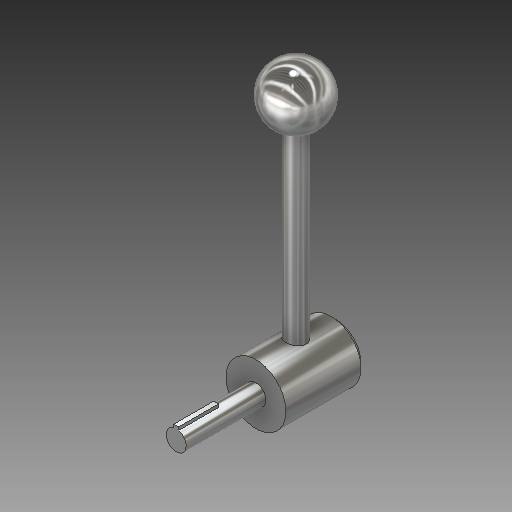
# Autodesk Inventor part: Handle
Saved by Autodesk Inventor 2018 (Build 220112000, 112)
## iProperties
Created: 2017-12-22
Part Number: Handle
Material: Stainless Steel
Document SubType Name: Modeling
Designer: 232963
Density: 8 g/cm^3
Appearance: Chrome - Polished
Author: 232963
Autodesk Inventor part; units mm, degrees
ref_plane "YZ Plane" through (0, 0, 0) normal (1, 0, 0) x (0, 1, 0)
ref_plane "XZ Plane" through (0, 0, 0) normal (0, 1, 0) x (-1, 0, 0)
ref_plane "XY Plane" through (0, 0, 0) normal (0, 0, 1) x (1, 0, 0)
sketch "Sketch1" plane through (0, 0, 0) normal (0, 0, 1) x (1, 0, 0)
  circle A0 centre (0, 0) radius 9.525
  dimension "d0" = 19.05
  constraints: 1 centre point, 1 coincident
  measures "d0" diameter of A0
extrude "Extrusion1" add sketch "Sketch1" along normal blind 25.4
sketch "Sketch2" plane through (0, 0, 25.4) normal (0, 0, 1) x (1, 0, 0)
  circle A0 centre (0, 0) radius 3.175
  dimension "d3" = 6.35
  constraints: 1 centre point, 1 coincident
  measures "d3" diameter of A0
extrude "Extrusion2" add sketch "Sketch2" along normal blind 25.4
sketch "Sketch3" plane through (0, 0, 50.8) normal (0, 0, 1) x (1, 0, 0)
  line L0 (-0.762, 4.064) -> (0.762, 4.064)
  line L1 (0.762, 4.064) -> (0.762, 2.2428)
  line L2 (0.762, 2.2428) -> (-0.762, 2.2428)
  line L3 (-0.762, 2.2428) -> (-0.762, 4.064)
  point P0 (0, 0)
  dimension "d6" = 4.064
  dimension "d7" = 0.762
  dimension "d8" = 1.524
  constraints: 8 end point, 2 parallel, 1 horizontal, 1 perpendicular
  measures "d6" distance from line of point (0, 0) L0
  measures "d7" distance from line of point (0, 0) L3
  measures "d8" distance of L0.start L0.end
extrude "Extrusion3" add sketch "Sketch3" against normal blind 12.7
sketch "Sketch4" plane through (0, 0, 0) normal (0, 1, 0) x (-1, 0, 0)
  line L0 (-9.525, 0) -> (-9.525, 25.4) projected
  line L1 (-9.525, 25.4) -> (-3.175, 25.4) projected
  line L2 (-3.175, 25.4) -> (-3.175, 50.8) projected
  line L3 (-3.175, 50.8) -> (3.175, 50.8) projected
  line L4 (3.175, 50.8) -> (3.175, 25.4) projected
  line L5 (3.175, 25.4) -> (9.525, 25.4) projected
  line L6 (9.525, 25.4) -> (9.525, 0) projected
  line L7 (9.525, 0) -> (-9.525, 0) projected
  circle A0 centre (0, 12.7) radius 3.175
  point P0 (0, 0)
  dimension "d11" = 6.35
  dimension "d12" = 12.7
  dimension "d13" = 9.525
  constraints: 1 centre point
  measures "d11" diameter of A0
  measures "d12" distance from line of L7 A0.centre
  measures "d13" distance from line of L6 A0.centre
extrude "Extrusion4" add sketch "Sketch4" along normal blind 76.2 contours A0
sketch "Sketch5" plane through (0, 76.2, 12.7) normal (0, 1, 0) x (1, 0, 0)
  arc A0 (9.525, 0) -> (-9.525, 0) centre (0, 0) ccw
  line L0 (-9.525, 0) -> (9.525, 0)
  line L1 (9.525, 12.7) -> (9.525, -12.7) projected
  point P0 (0, 12.7)
  dimension "d16" = 19.05
  constraints: 2 end point, 2 midpoint, 2 point on circle, 1 centre point
  measures "d16" diameter of A0
revolve "Revolution1" add sketch "Sketch5" angle 360 about axis through (-9.525, 76.2, 12.7) along (1, 0, 0)
chamfer "Chamfer1" distance 1.524 angle 45 1 edges at (-9.525, 0, 0)
body "Solid1"
